Autodesk Fusion 360 part; units mm, degrees
(part 19 of 20)
  spline S762 degree 3 poles (33.1646, -486.3279) (33.0435, -486.3377) (32.8055, -486.3569) (32.6209, -486.5079) (32.5302, -486.582) knots 0 0 0 0 0.035532 0.069798 0.069798 0.069798 0.069798
  spline S763 degree 3 poles (32.5302, -486.582) (32.4569, -486.6887) (32.2898, -486.9318) (32.2821, -487.2288) (32.2779, -487.3954) knots 0 0 0 0 0.038079 0.086792 0.086792 0.086792 0.086792
  line L588 (32.2779, -487.3954) -> (32.2779, -489.4998)
  line L589 (32.2779, -489.4998) -> (31.664, -489.4998)
  line L590 (31.664, -489.4998) -> (31.6639, -487.1464)
  spline S764 degree 3 poles (31.6639, -487.1464) (31.6615, -487.0244) (31.6572, -486.8076) (31.5575, -486.6162) (31.5139, -486.5325) knots 0 0 0 0 0.036008 0.063954 0.063954 0.063954 0.063954
  spline S765 degree 3 poles (31.5139, -486.5325) (31.4516, -486.473) (31.3154, -486.3426) (31.1258, -486.3331) (31.0227, -486.3279) knots 0 0 0 0 0.025037 0.054812 0.054812 0.054812 0.054812
  spline S766 degree 3 poles (31.0227, -486.3279) (30.938, -486.3336) (30.7685, -486.3449) (30.6185, -486.4245) (30.5435, -486.4643) knots 0 0 0 0 0.025173 0.050327 0.050327 0.050327 0.050327
  spline S767 degree 3 poles (30.5435, -486.4643) (30.4749, -486.516) (30.3346, -486.6216) (30.2618, -486.7816) (30.2246, -486.8634) knots 0 0 0 0 0.025339 0.051812 0.051812 0.051812 0.051812
  spline S768 degree 3 poles (30.2246, -486.8634) (30.1959, -486.9697) (30.1291, -487.2172) (30.127, -487.474) (30.1258, -487.6205) knots 0 0 0 0 0.032907 0.076633 0.076633 0.076633 0.076633
  line L591 (30.1258, -487.6205) -> (30.1258, -489.4998)
  line L592 (30.1258, -489.4998) -> (29.5119, -489.4998)
  line L593 (18.0828, -488.1801) -> (18.6967, -488.0982)
  spline S769 degree 3 poles (18.6967, -488.0982) (18.7321, -488.254) (18.7955, -488.533) (18.9765, -488.7531) (19.0565, -488.8503) knots 0 0 0 0 0.04711 0.084389 0.084389 0.084389 0.084389
  spline S770 degree 3 poles (19.0565, -488.8503) (19.1469, -488.9174) (19.3307, -489.054) (19.5593, -489.0716) (19.6756, -489.0805) knots 0 0 0 0 0.033049 0.06726 0.06726 0.06726 0.06726
  spline S771 degree 3 poles (19.6756, -489.0805) (19.814, -489.0683) (20.0891, -489.0441) (20.3016, -488.8679) (20.4071, -488.7803) knots 0 0 0 0 0.040646 0.080767 0.080767 0.080767 0.080767
  spline S772 degree 3 poles (20.4071, -488.7803) (20.4942, -488.6734) (20.6706, -488.4566) (20.6938, -488.1779) (20.7056, -488.0368) knots 0 0 0 0 0.040368 0.081802 0.081802 0.081802 0.081802
  spline S773 degree 3 poles (20.7056, -488.0368) (20.6952, -487.9031) (20.6748, -487.6418) (20.5099, -487.4386) (20.4293, -487.3393) knots 0 0 0 0 0.039196 0.07662 0.07662 0.07662 0.07662
  spline S774 degree 3 poles (20.4293, -487.3393) (20.3292, -487.2593) (20.1239, -487.095) (19.8613, -487.075) (19.7267, -487.0648) knots 0 0 0 0 0.037531 0.077014 0.077014 0.077014 0.077014
  spline S775 degree 3 poles (19.7267, -487.0648) (19.6613, -487.0687) (19.5148, -487.0774) (19.3724, -487.1132) (19.2935, -487.133) knots 0 0 0 0 0.0196 0.043933 0.043933 0.043933 0.043933
  line L594 (19.2935, -487.133) -> (19.3618, -486.5941)
  spline S776 degree 3 poles (19.3618, -486.5941) (19.3802, -486.5961) (19.4131, -486.5996) (19.4462, -486.6005) (19.4607, -486.6009) knots 0 0 0 0 0.005566 0.009918 0.009918 0.009918 0.009918
  spline S777 degree 3 poles (19.4607, -486.6009) (19.5875, -486.5928) (19.838, -486.5768) (20.058, -486.456) (20.1667, -486.3963) knots 0 0 0 0 0.037611 0.074313 0.074313 0.074313 0.074313
  spline S778 degree 3 poles (20.1667, -486.3963) (20.2581, -486.3162) (20.4485, -486.1497) (20.4695, -485.8967) (20.4804, -485.7653) knots 0 0 0 0 0.035073 0.072985 0.072985 0.072985 0.072985
  spline S779 degree 3 poles (20.4804, -485.7653) (20.4716, -485.6582) (20.4541, -485.4476) (20.3186, -485.2856) (20.2519, -485.206) knots 0 0 0 0 0.031391 0.061757 0.061757 0.061757 0.061757
  spline S780 degree 3 poles (20.2519, -485.206) (20.1682, -485.1413) (19.9946, -485.0073) (19.7754, -484.9921) (19.6619, -484.9843) knots 0 0 0 0 0.031011 0.064303 0.064303 0.064303 0.064303
  spline S781 degree 3 poles (19.6619, -484.9843) (19.5485, -484.9927) (19.3271, -485.0092) (19.1509, -485.1438) (19.065, -485.2094) knots 0 0 0 0 0.033306 0.06503 0.06503 0.06503 0.06503
  spline S782 degree 3 poles (19.065, -485.2094) (18.9918, -485.2995) (18.8312, -485.4971) (18.7838, -485.7481) (18.7581, -485.8847) knots 0 0 0 0 0.034298 0.07522 0.07522 0.07522 0.07522
  line L595 (18.7581, -485.8847) -> (18.1441, -485.7756)
  spline S783 degree 3 poles (18.1441, -485.7756) (18.19, -485.5845) (18.2776, -485.2203) (18.5339, -484.9482) (18.6557, -484.8189) knots 0 0 0 0 0.057796 0.110176 0.110176 0.110176 0.110176
  spline S784 degree 3 poles (18.6557, -484.8189) (18.8, -484.7199) (19.0988, -484.515) (19.461, -484.4916) (19.6482, -484.4795) knots 0 0 0 0 0.051494 0.106636 0.106636 0.106636 0.106636
  spline S785 degree 3 poles (19.6482, -484.4795) (19.7811, -484.4864) (20.0429, -484.4999) (20.2835, -484.6039) (20.402, -484.6551) knots 0 0 0 0 0.039552 0.07795 0.07795 0.07795 0.07795
  spline S786 degree 3 poles (20.402, -484.6551) (20.5093, -484.7178) (20.7191, -484.8402) (20.8601, -485.0378) (20.9289, -485.1343) knots 0 0 0 0 0.036811 0.071949 0.071949 0.071949 0.071949
  spline S787 degree 3 poles (20.9289, -485.1343) (20.9821, -485.2365) (21.0875, -485.4388) (21.1035, -485.6663) (21.1114, -485.7789) knots 0 0 0 0 0.034154 0.067635 0.067635 0.067635 0.067635
  spline S788 degree 3 poles (21.1114, -485.7789) (21.1043, -485.8843) (21.0902, -486.0939) (20.9882, -486.2776) (20.9375, -486.369) knots 0 0 0 0 0.031256 0.062193 0.062193 0.062193 0.062193
  spline S789 degree 3 poles (20.9375, -486.369) (20.8702, -486.4542) (20.7295, -486.6323) (20.5278, -486.7372) (20.4225, -486.7919) knots 0 0 0 0 0.032177 0.067318 0.067318 0.067318 0.067318
  spline S790 degree 3 poles (20.4225, -486.7919) (20.5606, -486.8334) (20.8284, -486.9138) (21.0191, -487.1178) (21.1114, -487.2165) knots 0 0 0 0 0.042418 0.082229 0.082229 0.082229 0.082229
  spline S791 degree 3 poles (21.1114, -487.2165) (21.183, -487.3343) (21.3334, -487.5817) (21.3489, -487.8713) (21.357, -488.0231) knots 0 0 0 0 0.040688 0.085491 0.085491 0.085491 0.085491
  spline S792 degree 3 poles (21.357, -488.0231) (21.3369, -488.2333) (21.2967, -488.6544) (21.0188, -488.9735) (20.8795, -489.1333) knots 0 0 0 0 0.061663 0.123588 0.123588 0.123588 0.123588
  spline S793 degree 3 poles (20.8795, -489.1333) (20.7066, -489.2661) (20.3507, -489.5393) (19.9026, -489.5719) (19.6722, -489.5886) knots 0 0 0 0 0.063941 0.131584 0.131584 0.131584 0.131584
  spline S794 degree 3 poles (19.6722, -489.5886) (19.4646, -489.5745) (19.0624, -489.5472) (18.7367, -489.3108) (18.5791, -489.1964) knots 0 0 0 0 0.061033 0.118246 0.118246 0.118246 0.118246
  spline S795 degree 3 poles (18.5791, -489.1964) (18.4495, -489.0541) (18.1853, -488.764) (18.1174, -488.3772) (18.0828, -488.1801) knots 0 0 0 0 0.056507 0.1152 0.1152 0.1152 0.1152
  line L596 (29.5184, -539.499) -> (29.5181, -535.8769)
  line L597 (29.5181, -535.8769) -> (30.0672, -535.8768)
  line L598 (30.0672, -535.8768) -> (30.0672, -536.385)
  spline S796 degree 3 poles (30.0672, -536.385) (30.1291, -536.3004) (30.254, -536.1299) (30.4314, -536.0149) (30.5208, -535.9569) knots 0 0 0 0 0.031158 0.062835 0.062835 0.062835 0.062835
  spline S797 degree 3 poles (30.5208, -535.9569) (30.62, -535.9097) (30.8239, -535.8125) (31.0495, -535.8009) (31.1654, -535.7949) knots 0 0 0 0 0.032617 0.067048 0.067048 0.067048 0.067048
  spline S798 degree 3 poles (31.1654, -535.7949) (31.2899, -535.7996) (31.5223, -535.8084) (31.7293, -535.9133) (31.8254, -535.9619) knots 0 0 0 0 0.036859 0.068796 0.068796 0.068796 0.068796
  spline S799 degree 3 poles (31.8254, -535.9619) (31.9051, -536.0236) (32.066, -536.1483) (32.1475, -536.3349) (32.1887, -536.4291) knots 0 0 0 0 0.029725 0.060035 0.060035 0.060035 0.060035
  spline S800 degree 3 poles (32.1887, -536.4291) (32.3388, -536.2442) (32.6299, -535.8856) (33.0863, -535.8243) (33.3073, -535.7947) knots 0 0 0 0 0.068625 0.133023 0.133023 0.133023 0.133023
  spline S801 degree 3 poles (33.3073, -535.7947) (33.4724, -535.8031) (33.7803, -535.8187) (34.0234, -536.0061) (34.1361, -536.093) knots 0 0 0 0 0.048244 0.08997 0.08997 0.08997 0.08997
  spline S802 degree 3 poles (34.1361, -536.093) (34.2204, -536.2154) (34.4099, -536.4902) (34.4203, -536.8259) (34.4261, -537.0122) knots 0 0 0 0 0.043695 0.098195 0.098195 0.098195 0.098195
  line L599 (34.4261, -537.0122) -> (34.4263, -539.4985)
  line L600 (34.4263, -539.4985) -> (33.8158, -539.4986)
  line L601 (33.8158, -539.4986) -> (33.8156, -537.2169)
  spline S803 degree 3 poles (33.8156, -537.2169) (33.8156, -537.1106) (33.8155, -536.9313) (33.7731, -536.7574) (33.7559, -536.6865) knots 0 0 0 0 0.031711 0.053535 0.053535 0.053535 0.053535
  spline S804 degree 3 poles (33.7559, -536.6865) (33.7314, -536.6348) (33.6816, -536.5294) (33.5873, -536.4607) (33.5393, -536.4256) knots 0 0 0 0 0.016863 0.034394 0.034394 0.034394 0.034394
  spline S805 degree 3 poles (33.5393, -536.4256) (33.4836, -536.3968) (33.3681, -536.337) (33.2381, -536.3303) (33.1709, -536.3267) knots 0 0 0 0 0.018597 0.038532 0.038532 0.038532 0.038532
  spline S806 degree 3 poles (33.1709, -536.3267) (33.0498, -536.3366) (32.8118, -536.3558) (32.6272, -536.5068) (32.5366, -536.5809) knots 0 0 0 0 0.035532 0.069798 0.069798 0.069798 0.069798
  spline S807 degree 3 poles (32.5366, -536.5809) (32.4632, -536.6876) (32.2961, -536.9308) (32.2885, -537.2277) (32.2842, -537.3944) knots 0 0 0 0 0.038079 0.086792 0.086792 0.086792 0.086792
  line L602 (32.2842, -537.3944) -> (32.2844, -539.4987)
  line L603 (32.2844, -539.4987) -> (31.6705, -539.4988)
  line L604 (31.6705, -539.4988) -> (31.6703, -537.1454)
  spline S808 degree 3 poles (31.6703, -537.1454) (31.6679, -537.0234) (31.6636, -536.8066) (31.5638, -536.6152) (31.5202, -536.5315) knots 0 0 0 0 0.036008 0.063954 0.063954 0.063954 0.063954
  spline S809 degree 3 poles (31.5202, -536.5315) (31.458, -536.472) (31.3217, -536.3416) (31.1321, -536.3321) (31.029, -536.3269) knots 0 0 0 0 0.025037 0.054812 0.054812 0.054812 0.054812
  spline S810 degree 3 poles (31.029, -536.3269) (30.9443, -536.3326) (30.7748, -536.344) (30.6248, -536.4236) (30.5499, -536.4634) knots 0 0 0 0 0.025173 0.050327 0.050327 0.050327 0.050327
  spline S811 degree 3 poles (30.5499, -536.4634) (30.4812, -536.5151) (30.3409, -536.6207) (30.2682, -536.7807) (30.231, -536.8625) knots 0 0 0 0 0.025339 0.051812 0.051812 0.051812 0.051812
  spline S812 degree 3 poles (30.231, -536.8625) (30.2023, -536.9688) (30.1355, -537.2163) (30.1334, -537.4731) (30.1321, -537.6196) knots 0 0 0 0 0.032907 0.076633 0.076633 0.076633 0.076633
  line L605 (30.1321, -537.6196) -> (30.1323, -539.4989)
  line L606 (30.1323, -539.4989) -> (29.5184, -539.499)
  line L607 (18.0892, -538.18) -> (18.7031, -538.0981)
  spline S813 degree 3 poles (18.7031, -538.0981) (18.7385, -538.2539) (18.8019, -538.5329) (18.983, -538.7529) (19.063, -538.8501) knots 0 0 0 0 0.04711 0.084389 0.084389 0.084389 0.084389
  spline S814 degree 3 poles (19.063, -538.8501) (19.1534, -538.9173) (19.3372, -539.0539) (19.5658, -539.0714) (19.6821, -539.0803) knots 0 0 0 0 0.033049 0.06726 0.06726 0.06726 0.06726
  spline S815 degree 3 poles (19.6821, -539.0803) (19.8205, -539.0681) (20.0956, -539.0439) (20.3081, -538.8676) (20.4136, -538.7801) knots 0 0 0 0 0.040646 0.080767 0.080767 0.080767 0.080767
  spline S816 degree 3 poles (20.4136, -538.7801) (20.5007, -538.6731) (20.677, -538.4564) (20.7002, -538.1777) (20.712, -538.0365) knots 0 0 0 0 0.040368 0.081802 0.081802 0.081802 0.081802
  spline S817 degree 3 poles (20.712, -538.0365) (20.7016, -537.9029) (20.6812, -537.6416) (20.5162, -537.4384) (20.4357, -537.3391) knots 0 0 0 0 0.039196 0.07662 0.07662 0.07662 0.07662
  spline S818 degree 3 poles (20.4357, -537.3391) (20.3356, -537.259) (20.1303, -537.0948) (19.8677, -537.0748) (19.7331, -537.0646) knots 0 0 0 0 0.037531 0.077014 0.077014 0.077014 0.077014
  spline S819 degree 3 poles (19.7331, -537.0646) (19.6677, -537.0685) (19.5212, -537.0772) (19.3788, -537.113) (19.2999, -537.1328) knots 0 0 0 0 0.0196 0.043933 0.043933 0.043933 0.043933
  line L608 (19.2999, -537.1328) -> (19.3681, -536.594)
  spline S820 degree 3 poles (19.3681, -536.594) (19.3865, -536.5959) (19.4194, -536.5995) (19.4525, -536.6004) (19.467, -536.6008) knots 0 0 0 0 0.005566 0.009918 0.009918 0.009918 0.009918
  spline S821 degree 3 poles (19.467, -536.6008) (19.5938, -536.5927) (19.8444, -536.5766) (20.0643, -536.4558) (20.173, -536.3961) knots 0 0 0 0 0.037611 0.074313 0.074313 0.074313 0.074313
  spline S822 degree 3 poles (20.173, -536.3961) (20.2644, -536.316) (20.4548, -536.1495) (20.4758, -535.8965) (20.4867, -535.7651) knots 0 0 0 0 0.035073 0.072985 0.072985 0.072985 0.072985
  spline S823 degree 3 poles (20.4867, -535.7651) (20.4778, -535.658) (20.4603, -535.4473) (20.3248, -535.2854) (20.2581, -535.2058) knots 0 0 0 0 0.031391 0.061757 0.061757 0.061757 0.061757
  spline S824 degree 3 poles (20.2581, -535.2058) (20.1744, -535.1411) (20.0008, -535.0071) (19.7816, -534.992) (19.6681, -534.9841) knots 0 0 0 0 0.031011 0.064303 0.064303 0.064303 0.064303
  spline S825 degree 3 poles (19.6681, -534.9841) (19.5547, -534.9926) (19.3333, -535.009) (19.1572, -535.1436) (19.0712, -535.2093) knots 0 0 0 0 0.033306 0.06503 0.06503 0.06503 0.06503
  spline S826 degree 3 poles (19.0712, -535.2093) (18.998, -535.2994) (18.8375, -535.4969) (18.7901, -535.748) (18.7643, -535.8846) knots 0 0 0 0 0.034298 0.07522 0.07522 0.07522 0.07522
  line L609 (18.7643, -535.8846) -> (18.1504, -535.7755)
  spline S827 degree 3 poles (18.1504, -535.7755) (18.1963, -535.5844) (18.2838, -535.2202) (18.5401, -534.9481) (18.6619, -534.8188) knots 0 0 0 0 0.057796 0.110176 0.110176 0.110176 0.110176
  spline S828 degree 3 poles (18.6619, -534.8188) (18.8062, -534.7198) (19.105, -534.5149) (19.4671, -534.4915) (19.6544, -534.4793) knots 0 0 0 0 0.051494 0.106636 0.106636 0.106636 0.106636
  spline S829 degree 3 poles (19.6544, -534.4793) (19.7872, -534.4862) (20.0491, -534.4997) (20.2896, -534.6037) (20.4082, -534.6549) knots 0 0 0 0 0.039552 0.07795 0.07795 0.07795 0.07795
  spline S830 degree 3 poles (20.4082, -534.6549) (20.5155, -534.7176) (20.7253, -534.84) (20.8663, -535.0376) (20.9351, -535.1341) knots 0 0 0 0 0.036811 0.071949 0.071949 0.071949 0.071949
  spline S831 degree 3 poles (20.9351, -535.1341) (20.9884, -535.2362) (21.0938, -535.4385) (21.1098, -535.6661) (21.1177, -535.7787) knots 0 0 0 0 0.034154 0.067635 0.067635 0.067635 0.067635
  spline S832 degree 3 poles (21.1177, -535.7787) (21.1106, -535.884) (21.0965, -536.0937) (20.9945, -536.2774) (20.9438, -536.3687) knots 0 0 0 0 0.031256 0.062193 0.062193 0.062193 0.062193
  spline S833 degree 3 poles (20.9438, -536.3687) (20.8765, -536.4539) (20.7358, -536.6321) (20.5341, -536.7369) (20.4288, -536.7917) knots 0 0 0 0 0.032177 0.067318 0.067318 0.067318 0.067318
  spline S834 degree 3 poles (20.4288, -536.7917) (20.567, -536.8332) (20.8348, -536.9135) (21.0255, -537.1175) (21.1178, -537.2163) knots 0 0 0 0 0.042418 0.082229 0.082229 0.082229 0.082229
  spline S835 degree 3 poles (21.1178, -537.2163) (21.1894, -537.334) (21.3398, -537.5814) (21.3553, -537.871) (21.3634, -538.0228) knots 0 0 0 0 0.040688 0.085491 0.085491 0.085491 0.085491
  spline S836 degree 3 poles (21.3634, -538.0228) (21.3434, -538.233) (21.3032, -538.6541) (21.0253, -538.9732) (20.886, -539.1331) knots 0 0 0 0 0.061663 0.123588 0.123588 0.123588 0.123588
  spline S837 degree 3 poles (20.886, -539.1331) (20.7131, -539.2658) (20.3573, -539.5391) (19.9091, -539.5717) (19.6787, -539.5885) knots 0 0 0 0 0.063941 0.131584 0.131584 0.131584 0.131584
  spline S838 degree 3 poles (19.6787, -539.5885) (19.4711, -539.5744) (19.0689, -539.547) (18.7432, -539.3107) (18.5856, -539.1963) knots 0 0 0 0 0.061033 0.118246 0.118246 0.118246 0.118246
  spline S839 degree 3 poles (18.5856, -539.1963) (18.456, -539.054) (18.1918, -538.7639) (18.1238, -538.3771) (18.0892, -538.18) knots 0 0 0 0 0.056507 0.1152 0.1152 0.1152 0.1152
  line L610 (29.5554, -589.4999) -> (29.5554, -585.8778)
  line L611 (29.5554, -585.8778) -> (30.1045, -585.8778)
  line L612 (30.1045, -585.8778) -> (30.1045, -586.386)
  spline S840 degree 3 poles (30.1045, -586.386) (30.1664, -586.3014) (30.2913, -586.1309) (30.4687, -586.0159) (30.5581, -585.958) knots 0 0 0 0 0.031158 0.062835 0.062835 0.062835 0.062835
  spline S841 degree 3 poles (30.5581, -585.958) (30.6573, -585.9107) (30.8612, -585.8136) (31.0868, -585.802) (31.2027, -585.796) knots 0 0 0 0 0.032617 0.067048 0.067048 0.067048 0.067048
  spline S842 degree 3 poles (31.2027, -585.796) (31.3272, -585.8007) (31.5596, -585.8095) (31.7666, -585.9144) (31.8627, -585.9631) knots 0 0 0 0 0.036859 0.068796 0.068796 0.068796 0.068796
  spline S843 degree 3 poles (31.8627, -585.9631) (31.9424, -586.0248) (32.1033, -586.1495) (32.1848, -586.3361) (32.2259, -586.4303) knots 0 0 0 0 0.029725 0.060035 0.060035 0.060035 0.060035
  spline S844 degree 3 poles (32.2259, -586.4303) (32.3761, -586.2454) (32.6672, -585.8868) (33.1236, -585.8256) (33.3446, -585.796) knots 0 0 0 0 0.068625 0.133023 0.133023 0.133023 0.133023
  spline S845 degree 3 poles (33.3446, -585.796) (33.5097, -585.8044) (33.8176, -585.82) (34.0607, -586.0075) (34.1734, -586.0944) knots 0 0 0 0 0.048244 0.08997 0.08997 0.08997 0.08997
  spline S846 degree 3 poles (34.1734, -586.0944) (34.2577, -586.2167) (34.4471, -586.4916) (34.4575, -586.8273) (34.4633, -587.0135) knots 0 0 0 0 0.043695 0.098195 0.098195 0.098195 0.098195
  line L613 (34.4633, -587.0135) -> (34.4633, -589.4999)
  line L614 (34.4633, -589.4999) -> (33.8528, -589.4999)
  line L615 (33.8528, -589.4999) -> (33.8528, -587.2182)
  spline S847 degree 3 poles (33.8528, -587.2182) (33.8528, -587.112) (33.8527, -586.9327) (33.8104, -586.7587) (33.7931, -586.6878) knots 0 0 0 0 0.031711 0.053535 0.053535 0.053535 0.053535
  spline S848 degree 3 poles (33.7931, -586.6878) (33.7687, -586.6362) (33.7188, -586.5308) (33.6246, -586.462) (33.5765, -586.4269) knots 0 0 0 0 0.016863 0.034394 0.034394 0.034394 0.034394
  spline S849 degree 3 poles (33.5765, -586.4269) (33.5208, -586.3981) (33.4054, -586.3383) (33.2754, -586.3315) (33.2082, -586.328) knots 0 0 0 0 0.018597 0.038532 0.038532 0.038532 0.038532
  spline S850 degree 3 poles (33.2082, -586.328) (33.087, -586.3378) (32.8491, -586.3571) (32.6644, -586.508) (32.5738, -586.5821) knots 0 0 0 0 0.035532 0.069798 0.069798 0.069798 0.069798
  spline S851 degree 3 poles (32.5738, -586.5821) (32.5005, -586.6888) (32.3333, -586.932) (32.3257, -587.2289) (32.3214, -587.3955) knots 0 0 0 0 0.038079 0.086792 0.086792 0.086792 0.086792
  line L616 (32.3214, -587.3955) -> (32.3214, -589.4999)
  line L617 (32.3214, -589.4999) -> (31.7075, -589.4999)
  line L618 (31.7075, -589.4999) -> (31.7075, -587.1466)
  spline S852 degree 3 poles (31.7075, -587.1466) (31.7051, -587.0245) (31.7008, -586.8077) (31.601, -586.6163) (31.5574, -586.5327) knots 0 0 0 0 0.036008 0.063954 0.063954 0.063954 0.063954
  spline S853 degree 3 poles (31.5574, -586.5327) (31.4952, -586.4731) (31.359, -586.3427) (31.1693, -586.3332) (31.0663, -586.328) knots 0 0 0 0 0.025037 0.054812 0.054812 0.054812 0.054812
  spline S854 degree 3 poles (31.0663, -586.328) (30.9815, -586.3337) (30.8121, -586.345) (30.6621, -586.4247) (30.5871, -586.4645) knots 0 0 0 0 0.025172 0.050327 0.050327 0.050327 0.050327
  spline S855 degree 3 poles (30.5871, -586.4645) (30.5185, -586.5161) (30.3782, -586.6217) (30.3054, -586.7817) (30.2682, -586.8635) knots 0 0 0 0 0.025339 0.051812 0.051812 0.051812 0.051812
  spline S856 degree 3 poles (30.2682, -586.8635) (30.2395, -586.9698) (30.1727, -587.2173) (30.1705, -587.4741) (30.1693, -587.6207) knots 0 0 0 0 0.032907 0.076633 0.076633 0.076633 0.076633
  line L619 (30.1693, -587.6207) -> (30.1693, -589.4999)
  line L620 (30.1693, -589.4999) -> (29.5554, -589.4999)
  line L621 (21.3494, -588.9099) -> (21.3494, -589.5)
  line L622 (21.3494, -589.5) -> (18.0445, -589.5)
  spline S857 degree 3 poles (18.0445, -589.5) (18.0457, -589.4269) (18.0482, -589.2812) (18.0935, -589.1427) (18.1161, -589.0737) knots 0 0 0 0 0.021791 0.043448 0.043448 0.043448 0.043448
  spline S858 degree 3 poles (18.1161, -589.0737) (18.1664, -588.9593) (18.2717, -588.7199) (18.435, -588.5154) (18.5203, -588.4086) knots 0 0 0 0 0.037314 0.078118 0.078118 0.078118 0.078118
  spline S859 degree 3 poles (18.5203, -588.4086) (18.6313, -588.2886) (18.8818, -588.0181) (19.1656, -587.7825) (19.3235, -587.6514) knots 0 0 0 0 0.048996 0.110487 0.110487 0.110487 0.110487
  spline S860 degree 3 poles (19.3235, -587.6514) (19.5582, -587.459) (19.9537, -587.1347) (20.2889, -586.7491) (20.4251, -586.5924) knots 0 0 0 0 0.090844 0.153043 0.153043 0.153043 0.153043
  spline S861 degree 3 poles (20.4251, -586.5924) (20.5085, -586.4701) (20.6616, -586.2455) (20.696, -585.9766) (20.7116, -585.854) knots 0 0 0 0 0.043642 0.080205 0.080205 0.080205 0.080205
  spline S862 degree 3 poles (20.7116, -585.854) (20.7008, -585.7372) (20.6793, -585.5042) (20.5268, -585.3268) (20.4507, -585.2384) knots 0 0 0 0 0.034264 0.068363 0.068363 0.068363 0.068363
  spline S863 degree 3 poles (20.4507, -585.2384) (20.3544, -585.1653) (20.1536, -585.0129) (19.9015, -584.9963) (19.7702, -584.9877) knots 0 0 0 0 0.035452 0.073952 0.073952 0.073952 0.073952
  spline S864 degree 3 poles (19.7702, -584.9877) (19.6321, -584.9966) (19.368, -585.0136) (19.16, -585.1762) (19.0608, -585.2537) knots 0 0 0 0 0.040455 0.077352 0.077352 0.077352 0.077352
  spline S865 degree 3 poles (19.0608, -585.2537) (18.9832, -585.3553) (18.8174, -585.572) (18.8004, -585.8453) (18.7914, -585.9904) knots 0 0 0 0 0.037518 0.080034 0.080034 0.080034 0.080034
  line L623 (18.7914, -585.9904) -> (18.1604, -585.9256)
  spline S866 degree 3 poles (18.1604, -585.9256) (18.1919, -585.7089) (18.2511, -585.3018) (18.5216, -584.9937) (18.6481, -584.8496) knots 0 0 0 0 0.064088 0.120417 0.120417 0.120417 0.120417
  spline S867 degree 3 poles (18.6481, -584.8496) (18.8081, -584.7418) (19.1503, -584.5111) (19.5637, -584.4905) (19.7839, -584.4795) knots 0 0 0 0 0.056784 0.121484 0.121484 0.121484 0.121484
  spline S868 degree 3 poles (19.7839, -584.4795) (20.0064, -584.4917) (20.4261, -584.5148) (20.7642, -584.7623) (20.923, -584.8786) knots 0 0 0 0 0.065229 0.123034 0.123034 0.123034 0.123034
  spline S869 degree 3 poles (20.923, -584.8786) (21.0454, -585.02) (21.2914, -585.3046) (21.3255, -585.6793) (21.3426, -585.8676) knots 0 0 0 0 0.054646 0.10988 0.10988 0.10988 0.10988
  spline S870 degree 3 poles (21.3426, -585.8676) (21.3372, -585.9678) (21.3263, -586.1707) (21.2556, -586.3612) (21.2198, -586.4577) knots 0 0 0 0 0.029916 0.060578 0.060578 0.060578 0.060578
  spline S871 degree 3 poles (21.2198, -586.4577) (21.1689, -586.5592) (21.0584, -586.7794) (20.8984, -586.967) (20.8122, -587.0682) knots 0 0 0 0 0.033943 0.073642 0.073642 0.073642 0.073642
  spline S872 degree 3 poles (20.8122, -587.0682) (20.6875, -587.1967) (20.3873, -587.5062) (20.0582, -587.7851) (19.8658, -587.9481) knots 0 0 0 0 0.05369 0.129298 0.129298 0.129298 0.129298
  spline S873 degree 3 poles (19.8658, -587.9481) (19.7127, -588.0758) (19.4698, -588.2784) (19.241, -588.4967) (19.1563, -588.5774) knots 0 0 0 0 0.059772 0.09485 0.09485 0.09485 0.09485
  spline S874 degree 3 poles (19.1563, -588.5774) (19.107, -588.6315) (19.012, -588.7356) (18.9345, -588.8533) (18.8971, -588.9099) knots 0 0 0 0 0.021914 0.042221 0.042221 0.042221 0.042221
  line L624 (18.8971, -588.9099) -> (21.3494, -588.9099)
  line L625 (29.5579, -639.4997) -> (29.5578, -635.8776)
  line L626 (29.5578, -635.8776) -> (30.1069, -635.8775)
  line L627 (30.1069, -635.8775) -> (30.1069, -636.3857)
  spline S875 degree 3 poles (30.1069, -636.3857) (30.1688, -636.3012) (30.2937, -636.1306) (30.4711, -636.0156) (30.5605, -635.9577) knots 0 0 0 0 0.031158 0.062835 0.062835 0.062835 0.062835
  spline S876 degree 3 poles (30.5605, -635.9577) (30.6597, -635.9104) (30.8636, -635.8133) (31.0892, -635.8016) (31.2051, -635.7956) knots 0 0 0 0 0.032617 0.067048 0.067048 0.067048 0.067048
  spline S877 degree 3 poles (31.2051, -635.7956) (31.3296, -635.8004) (31.562, -635.8092) (31.769, -635.9141) (31.8651, -635.9628) knots 0 0 0 0 0.036859 0.068796 0.068796 0.068796 0.068796
  spline S878 degree 3 poles (31.8651, -635.9628) (31.9448, -636.0245) (32.1057, -636.1491) (32.1872, -636.3358) (32.2283, -636.43) knots 0 0 0 0 0.029725 0.060035 0.060035 0.060035 0.060035
  spline S879 degree 3 poles (32.2283, -636.43) (32.3785, -636.245) (32.6696, -635.8865) (33.126, -635.8252) (33.347, -635.7956) knots 0 0 0 0 0.068625 0.133023 0.133023 0.133023 0.133023
  spline S880 degree 3 poles (33.347, -635.7956) (33.5121, -635.804) (33.82, -635.8197) (34.0631, -636.0071) (34.1758, -636.094) knots 0 0 0 0 0.048244 0.08997 0.08997 0.08997 0.08997
  spline S881 degree 3 poles (34.1758, -636.094) (34.2601, -636.2163) (34.4495, -636.4912) (34.4599, -636.8269) (34.4657, -637.0132) knots 0 0 0 0 0.043695 0.098195 0.098195 0.098195 0.098195
  line L628 (34.4657, -637.0132) -> (34.4658, -639.4995)
  line L629 (34.4658, -639.4995) -> (33.8553, -639.4995)
  line L630 (33.8553, -639.4995) -> (33.8552, -637.2178)
  spline S882 degree 3 poles (33.8552, -637.2178) (33.8552, -637.1116) (33.8552, -636.9323) (33.8128, -636.7584) (33.7955, -636.6875) knots 0 0 0 0 0.031711 0.053535 0.053535 0.053535 0.053535
  spline S883 degree 3 poles (33.7955, -636.6875) (33.7711, -636.6358) (33.7212, -636.5304) (33.627, -636.4616) (33.5789, -636.4266) knots 0 0 0 0 0.016863 0.034394 0.034394 0.034394 0.034394
  spline S884 degree 3 poles (33.5789, -636.4266) (33.5232, -636.3977) (33.4078, -636.338) (33.2778, -636.3312) (33.2106, -636.3277) knots 0 0 0 0 0.018597 0.038532 0.038532 0.038532 0.038532
  spline S885 degree 3 poles (33.2106, -636.3277) (33.0895, -636.3375) (32.8515, -636.3567) (32.6669, -636.5077) (32.5762, -636.5818) knots 0 0 0 0 0.035532 0.069798 0.069798 0.069798 0.069798
  spline S886 degree 3 poles (32.5762, -636.5818) (32.5029, -636.6885) (32.3358, -636.9316) (32.3281, -637.2286) (32.3239, -637.3952) knots 0 0 0 0 0.038079 0.086792 0.086792 0.086792 0.086792
  line L631 (32.3239, -637.3952) -> (32.3239, -639.4996)
  line L632 (32.3239, -639.4996) -> (31.71, -639.4996)
  line L633 (31.71, -639.4996) -> (31.7099, -637.1462)
  spline S887 degree 3 poles (31.7099, -637.1462) (31.7075, -637.0242) (31.7032, -636.8074) (31.6034, -636.616) (31.5598, -636.5323) knots 0 0 0 0 0.036008 0.063954 0.063954 0.063954 0.063954
  spline S888 degree 3 poles (31.5598, -636.5323) (31.4976, -636.4728) (31.3614, -636.3424) (31.1717, -636.3329) (31.0687, -636.3277) knots 0 0 0 0 0.025037 0.054812 0.054812 0.054812 0.054812
  spline S889 degree 3 poles (31.0687, -636.3277) (30.984, -636.3334) (30.8145, -636.3447) (30.6645, -636.4244) (30.5895, -636.4642) knots 0 0 0 0 0.025172 0.050327 0.050327 0.050327 0.050327
  spline S890 degree 3 poles (30.5895, -636.4642) (30.5209, -636.5158) (30.3806, -636.6214) (30.3078, -636.7814) (30.2706, -636.8632) knots 0 0 0 0 0.025339 0.051812 0.051812 0.051812 0.051812
  spline S891 degree 3 poles (30.2706, -636.8632) (30.2419, -636.9695) (30.1751, -637.2171) (30.173, -637.4738) (30.1717, -637.6204) knots 0 0 0 0 0.032907 0.076633 0.076633 0.076633 0.076633
  line L634 (30.1717, -637.6204) -> (30.1718, -639.4996)
  line L635 (30.1718, -639.4996) -> (29.5579, -639.4997)
  line L636 (21.3519, -638.9098) -> (21.3519, -639.4999)
  line L637 (21.3519, -639.4999) -> (18.047, -639.5)
  spline S892 degree 3 poles (18.047, -639.5) (18.0482, -639.4269) (18.0507, -639.2812) (18.096, -639.1427) (18.1186, -639.0736) knots 0 0 0 0 0.021791 0.043448 0.043448 0.043448 0.043448
  spline S893 degree 3 poles (18.1186, -639.0736) (18.1689, -638.9593) (18.2742, -638.7199) (18.4374, -638.5154) (18.5227, -638.4086) knots 0 0 0 0 0.037314 0.078118 0.078118 0.078118 0.078118
  spline S894 degree 3 poles (18.5227, -638.4086) (18.6338, -638.2886) (18.8843, -638.0181) (19.168, -637.7825) (19.3259, -637.6514) knots 0 0 0 0 0.048996 0.110487 0.110487 0.110487 0.110487
  spline S895 degree 3 poles (19.3259, -637.6514) (19.5606, -637.4589) (19.9561, -637.1347) (20.2913, -636.7491) (20.4275, -636.5923) knots 0 0 0 0 0.090844 0.153043 0.153043 0.153043 0.153043
  spline S896 degree 3 poles (20.4275, -636.5923) (20.5109, -636.4701) (20.6641, -636.2454) (20.6984, -635.9765) (20.714, -635.8539) knots 0 0 0 0 0.043642 0.080205 0.080205 0.080205 0.080205
  spline S897 degree 3 poles (20.714, -635.8539) (20.7032, -635.7371) (20.6817, -635.5041) (20.5292, -635.3268) (20.4531, -635.2383) knots 0 0 0 0 0.034264 0.068363 0.068363 0.068363 0.068363
  spline S898 degree 3 poles (20.4531, -635.2383) (20.3568, -635.1652) (20.156, -635.0128) (19.9039, -634.9963) (19.7726, -634.9876) knots 0 0 0 0 0.035452 0.073952 0.073952 0.073952 0.073952
  spline S899 degree 3 poles (19.7726, -634.9876) (19.6345, -634.9965) (19.3704, -635.0136) (19.1624, -635.1761) (19.0632, -635.2537) knots 0 0 0 0 0.040455 0.077352 0.077352 0.077352 0.077352
  spline S900 degree 3 poles (19.0632, -635.2537) (18.9855, -635.3553) (18.8198, -635.572) (18.8028, -635.8452) (18.7938, -635.9904) knots 0 0 0 0 0.037518 0.080034 0.080034 0.080034 0.080034
  line L638 (18.7938, -635.9904) -> (18.1628, -635.9256)
  spline S901 degree 3 poles (18.1628, -635.9256) (18.1943, -635.7089) (18.2535, -635.3018) (18.524, -634.9937) (18.6505, -634.8495) knots 0 0 0 0 0.064088 0.120417 0.120417 0.120417 0.120417
  spline S902 degree 3 poles (18.6505, -634.8495) (18.8105, -634.7417) (19.1526, -634.5111) (19.5661, -634.4904) (19.7863, -634.4795) knots 0 0 0 0 0.056784 0.121484 0.121484 0.121484 0.121484
  spline S903 degree 3 poles (19.7863, -634.4795) (20.0088, -634.4917) (20.4285, -634.5147) (20.7666, -634.7622) (20.9254, -634.8785) knots 0 0 0 0 0.065229 0.123034 0.123034 0.123034 0.123034
  spline S904 degree 3 poles (20.9254, -634.8785) (21.0478, -635.02) (21.2938, -635.3045) (21.3278, -635.6792) (21.345, -635.8675) knots 0 0 0 0 0.054646 0.10988 0.10988 0.10988 0.10988
  spline S905 degree 3 poles (21.345, -635.8675) (21.3396, -635.9677) (21.3287, -636.1706) (21.258, -636.3612) (21.2222, -636.4576) knots 0 0 0 0 0.029916 0.060578 0.060578 0.060578 0.060578
  spline S906 degree 3 poles (21.2222, -636.4576) (21.1713, -636.5591) (21.0608, -636.7793) (20.9009, -636.9669) (20.8146, -637.0681) knots 0 0 0 0 0.033943 0.073642 0.073642 0.073642 0.073642
  spline S907 degree 3 poles (20.8146, -637.0681) (20.69, -637.1966) (20.3897, -637.5062) (20.0606, -637.785) (19.8682, -637.9481) knots 0 0 0 0 0.05369 0.129298 0.129298 0.129298 0.129298
  spline S908 degree 3 poles (19.8682, -637.9481) (19.7151, -638.0758) (19.4723, -638.2784) (19.2434, -638.4966) (19.1588, -638.5774) knots 0 0 0 0 0.059772 0.09485 0.09485 0.09485 0.09485
  spline S909 degree 3 poles (19.1588, -638.5774) (19.1095, -638.6314) (19.0145, -638.7356) (18.9369, -638.8533) (18.8996, -638.9099) knots 0 0 0 0 0.021914 0.042221 0.042221 0.042221 0.042221
  line L639 (18.8996, -638.9099) -> (21.3519, -638.9098)
  line L640 (29.2783, -689.4998) -> (29.2783, -685.8777)
  line L641 (29.2783, -685.8777) -> (29.8274, -685.8777)
  line L642 (29.8274, -685.8777) -> (29.8274, -686.3859)
  spline S910 degree 3 poles (29.8274, -686.3859) (29.8893, -686.3014) (30.0142, -686.1308) (30.1916, -686.0158) (30.281, -685.9579) knots 0 0 0 0 0.031158 0.062835 0.062835 0.062835 0.062835
  spline S911 degree 3 poles (30.281, -685.9579) (30.3802, -685.9106) (30.5841, -685.8135) (30.8097, -685.8019) (30.9256, -685.7959) knots 0 0 0 0 0.032617 0.067048 0.067048 0.067048 0.067048
  spline S912 degree 3 poles (30.9256, -685.7959) (31.0501, -685.8006) (31.2825, -685.8095) (31.4895, -685.9143) (31.5856, -685.963) knots 0 0 0 0 0.036859 0.068796 0.068796 0.068796 0.068796
  spline S913 degree 3 poles (31.5856, -685.963) (31.6652, -686.0247) (31.8262, -686.1494) (31.9077, -686.336) (31.9488, -686.4302) knots 0 0 0 0 0.029725 0.060035 0.060035 0.060035 0.060035
  spline S914 degree 3 poles (31.9488, -686.4302) (32.099, -686.2453) (32.3901, -685.8867) (32.8465, -685.8255) (33.0675, -685.7958) knots 0 0 0 0 0.068625 0.133023 0.133023 0.133023 0.133023
  spline S915 degree 3 poles (33.0675, -685.7958) (33.2326, -685.8042) (33.5405, -685.8199) (33.7835, -686.0073) (33.8963, -686.0943) knots 0 0 0 0 0.048244 0.08997 0.08997 0.08997 0.08997
  spline S916 degree 3 poles (33.8963, -686.0943) (33.9806, -686.2166) (34.17, -686.4915) (34.1804, -686.8271) (34.1862, -687.0134) knots 0 0 0 0 0.043695 0.098195 0.098195 0.098195 0.098195
  line L643 (34.1862, -687.0134) -> (34.1862, -689.4998)
  line L644 (34.1862, -689.4998) -> (33.5757, -689.4998)
  line L645 (33.5757, -689.4998) -> (33.5757, -687.2181)
  spline S917 degree 3 poles (33.5757, -687.2181) (33.5757, -687.1119) (33.5756, -686.9325) (33.5333, -686.7586) (33.516, -686.6877) knots 0 0 0 0 0.031711 0.053535 0.053535 0.053535 0.053535
  spline S918 degree 3 poles (33.516, -686.6877) (33.4916, -686.636) (33.4417, -686.5306) (33.3475, -686.4619) (33.2994, -686.4268) knots 0 0 0 0 0.016863 0.034394 0.034394 0.034394 0.034394
  spline S919 degree 3 poles (33.2994, -686.4268) (33.2437, -686.398) (33.1283, -686.3382) (32.9983, -686.3314) (32.9311, -686.3279) knots 0 0 0 0 0.018597 0.038532 0.038532 0.038532 0.038532
  spline S920 degree 3 poles (32.9311, -686.3279) (32.8099, -686.3377) (32.572, -686.357) (32.3873, -686.5079) (32.2967, -686.582) knots 0 0 0 0 0.035532 0.069798 0.069798 0.069798 0.069798
  spline S921 degree 3 poles (32.2967, -686.582) (32.2234, -686.6887) (32.0562, -686.9319) (32.0486, -687.2288) (32.0443, -687.3954) knots 0 0 0 0 0.038079 0.086792 0.086792 0.086792 0.086792
  line L646 (32.0443, -687.3954) -> (32.0443, -689.4998)
  line L647 (32.0443, -689.4998) -> (31.4304, -689.4998)
  line L648 (31.4304, -689.4998) -> (31.4304, -687.1465)
  spline S922 degree 3 poles (31.4304, -687.1465) (31.428, -687.0244) (31.4237, -686.8076) (31.3239, -686.6162) (31.2803, -686.5326) knots 0 0 0 0 0.036008 0.063954 0.063954 0.063954 0.063954
  spline S923 degree 3 poles (31.2803, -686.5326) (31.2181, -686.473) (31.0819, -686.3426) (30.8922, -686.3331) (30.7892, -686.3279) knots 0 0 0 0 0.025037 0.054812 0.054812 0.054812 0.054812
  spline S924 degree 3 poles (30.7892, -686.3279) (30.7044, -686.3336) (30.535, -686.345) (30.385, -686.4246) (30.31, -686.4644) knots 0 0 0 0 0.025173 0.050327 0.050327 0.050327 0.050327
  spline S925 degree 3 poles (30.31, -686.4644) (30.2414, -686.516) (30.1011, -686.6216) (30.0283, -686.7817) (29.9911, -686.8634) knots 0 0 0 0 0.025339 0.051812 0.051812 0.051812 0.051812
  spline S926 degree 3 poles (29.9911, -686.8634) (29.9624, -686.9697) (29.8956, -687.2173) (29.8934, -687.474) (29.8922, -687.6206) knots 0 0 0 0 0.032907 0.076633 0.076633 0.076633 0.076633
  line L649 (29.8922, -687.6206) -> (29.8922, -689.4998)
  line L650 (29.8922, -689.4998) -> (29.2783, -689.4998)
  line L651 (20.1583, -689.5) -> (19.5443, -689.5)
  line L652 (19.5443, -689.5) -> (19.5443, -685.588)
  spline S927 degree 3 poles (19.5443, -685.588) (19.4606, -685.6608) (19.2792, -685.8187) (19.0736, -685.9436) (18.9628, -686.0109) knots 0 0 0 0 0.033221 0.072019 0.072019 0.072019 0.072019
  spline S928 degree 3 poles (18.9628, -686.0109) (18.8503, -686.0753) (18.6416, -686.1948) (18.4191, -686.286) (18.3165, -686.3281) knots 0 0 0 0 0.03884 0.072064 0.072064 0.072064 0.072064
  line L653 (18.3165, -686.3281) -> (18.3165, -685.7346)
  spline S929 degree 3 poles (18.3165, -685.7346) (18.4811, -685.6511) (18.8025, -685.4881) (19.081, -685.2595) (19.2169, -685.148) knots 0 0 0 0 0.05519 0.10775 0.10775 0.10775 0.10775
  spline S930 degree 3 poles (19.2169, -685.148) (19.3329, -685.0399) (19.5456, -684.8418) (19.6947, -684.5927) (19.7626, -684.4795) knots 0 0 0 0 0.047275 0.086674 0.086674 0.086674 0.086674
  line L654 (19.7626, -684.4795) -> (20.1582, -684.4795)
  line L655 (20.1582, -684.4795) -> (20.1583, -689.5)
  line L656 (29.2799, -739.4997) -> (29.2798, -735.8776)
  line L657 (29.2798, -735.8776) -> (29.8289, -735.8776)
  line L658 (29.8289, -735.8776) -> (29.8289, -736.3858)
  spline S931 degree 3 poles (29.8289, -736.3858) (29.8908, -736.3012) (30.0157, -736.1307) (30.1931, -736.0157) (30.2825, -735.9577) knots 0 0 0 0 0.031158 0.062835 0.062835 0.062835 0.062835
  spline S932 degree 3 poles (30.2825, -735.9577) (30.3817, -735.9105) (30.5856, -735.8134) (30.8112, -735.8017) (30.9271, -735.7957) knots 0 0 0 0 0.032617 0.067048 0.067048 0.067048 0.067048
  spline S933 degree 3 poles (30.9271, -735.7957) (31.0516, -735.8004) (31.284, -735.8093) (31.491, -735.9141) (31.5871, -735.9628) knots 0 0 0 0 0.036859 0.068796 0.068796 0.068796 0.068796
  spline S934 degree 3 poles (31.5871, -735.9628) (31.6668, -736.0245) (31.8277, -736.1492) (31.9092, -736.3358) (31.9503, -736.4301) knots 0 0 0 0 0.029725 0.060035 0.060035 0.060035 0.060035
  spline S935 degree 3 poles (31.9503, -736.4301) (32.1005, -736.2451) (32.3916, -735.8865) (32.848, -735.8253) (33.069, -735.7957) knots 0 0 0 0 0.068625 0.133023 0.133023 0.133023 0.133023
  spline S936 degree 3 poles (33.069, -735.7957) (33.2341, -735.8041) (33.542, -735.8197) (33.7851, -736.0072) (33.8978, -736.0941) knots 0 0 0 0 0.048244 0.08997 0.08997 0.08997 0.08997
  spline S937 degree 3 poles (33.8978, -736.0941) (33.9821, -736.2164) (34.1715, -736.4913) (34.1819, -736.8269) (34.1877, -737.0132) knots 0 0 0 0 0.043695 0.098195 0.098195 0.098195 0.098195
  line L659 (34.1877, -737.0132) -> (34.1878, -739.4996)
  line L660 (34.1878, -739.4996) -> (33.5773, -739.4996)
  line L661 (33.5773, -739.4996) -> (33.5772, -737.2179)
  spline S938 degree 3 poles (33.5772, -737.2179) (33.5772, -737.1117) (33.5772, -736.9323) (33.5348, -736.7584) (33.5175, -736.6875) knots 0 0 0 0 0.031711 0.053535 0.053535 0.053535 0.053535
  spline S939 degree 3 poles (33.5175, -736.6875) (33.4931, -736.6359) (33.4432, -736.5305) (33.349, -736.4617) (33.3009, -736.4266) knots 0 0 0 0 0.016863 0.034394 0.034394 0.034394 0.034394
  spline S940 degree 3 poles (33.3009, -736.4266) (33.2452, -736.3978) (33.1298, -736.338) (32.9998, -736.3312) (32.9326, -736.3277) knots 0 0 0 0 0.018597 0.038532 0.038532 0.038532 0.038532
  spline S941 degree 3 poles (32.9326, -736.3277) (32.8115, -736.3375) (32.5735, -736.3568) (32.3889, -736.5077) (32.2982, -736.5818) knots 0 0 0 0 0.035532 0.069798 0.069798 0.069798 0.069798
  spline S942 degree 3 poles (32.2982, -736.5818) (32.2249, -736.6885) (32.0578, -736.9317) (32.0501, -737.2286) (32.0459, -737.3953) knots 0 0 0 0 0.038079 0.086792 0.086792 0.086792 0.086792
  line L662 (32.0459, -737.3953) -> (32.0459, -739.4996)
  line L663 (32.0459, -739.4996) -> (31.432, -739.4997)
  line L664 (31.432, -739.4997) -> (31.4319, -737.1463)
  spline S943 degree 3 poles (31.4319, -737.1463) (31.4295, -737.0243) (31.4252, -736.8075) (31.3254, -736.6161) (31.2818, -736.5324) knots 0 0 0 0 0.036008 0.063954 0.063954 0.063954 0.063954
  spline S944 degree 3 poles (31.2818, -736.5324) (31.2196, -736.4728) (31.0834, -736.3424) (30.8937, -736.3329) (30.7907, -736.3278) knots 0 0 0 0 0.025037 0.054812 0.054812 0.054812 0.054812
  spline S945 degree 3 poles (30.7907, -736.3278) (30.706, -736.3335) (30.5365, -736.3448) (30.3865, -736.4244) (30.3115, -736.4642) knots 0 0 0 0 0.025172 0.050327 0.050327 0.050327 0.050327
  spline S946 degree 3 poles (30.3115, -736.4642) (30.2429, -736.5159) (30.1026, -736.6215) (30.0298, -736.7815) (29.9926, -736.8633) knots 0 0 0 0 0.025339 0.051812 0.051812 0.051812 0.051812
  spline S947 degree 3 poles (29.9926, -736.8633) (29.9639, -736.9696) (29.8971, -737.2171) (29.895, -737.4739) (29.8937, -737.6204) knots 0 0 0 0 0.032907 0.076633 0.076633 0.076633 0.076633
  line L665 (29.8937, -737.6204) -> (29.8938, -739.4997)
  line L666 (29.8938, -739.4997) -> (29.2799, -739.4997)
  line L667 (20.1598, -739.4999) -> (19.5459, -739.4999)
  line L668 (19.5459, -739.4999) -> (19.5458, -735.5879)
  spline S948 degree 3 poles (19.5458, -735.5879) (19.4621, -735.6608) (19.2807, -735.8186) (19.0751, -735.9436) (18.9643, -736.0109) knots 0 0 0 0 0.033221 0.072019 0.072019 0.072019 0.072019
  spline S949 degree 3 poles (18.9643, -736.0109) (18.8518, -736.0753) (18.6431, -736.1948) (18.4206, -736.286) (18.318, -736.3281) knots 0 0 0 0 0.03884 0.072064 0.072064 0.072064 0.072064
  line L669 (18.318, -736.3281) -> (18.318, -735.7346)
  spline S950 degree 3 poles (18.318, -735.7346) (18.4826, -735.6511) (18.804, -735.488) (19.0825, -735.2595) (19.2184, -735.148) knots 0 0 0 0 0.05519 0.10775 0.10775 0.10775 0.10775
  spline S951 degree 3 poles (19.2184, -735.148) (19.3344, -735.0399) (19.5471, -734.8418) (19.6962, -734.5927) (19.7641, -734.4795) knots 0 0 0 0 0.047275 0.086674 0.086674 0.086674 0.086674
  line L670 (19.7641, -734.4795) -> (20.1597, -734.4795)
  line L671 (20.1597, -734.4795) -> (20.1598, -739.4999)
  line L672 (28.5502, -789.465) -> (28.5499, -785.8429)
  line L673 (28.5499, -785.8429) -> (29.0991, -785.8429)
  line L674 (29.0991, -785.8429) -> (29.0991, -786.3511)
  spline S952 degree 3 poles (29.0991, -786.3511) (29.161, -786.2665) (29.2859, -786.096) (29.4633, -785.981) (29.5527, -785.923) knots 0 0 0 0 0.031158 0.062835 0.062835 0.062835 0.062835
  spline S953 degree 3 poles (29.5527, -785.923) (29.6519, -785.8758) (29.8557, -785.7786) (30.0814, -785.767) (30.1973, -785.761) knots 0 0 0 0 0.032617 0.067048 0.067048 0.067048 0.067048
  spline S954 degree 3 poles (30.1973, -785.761) (30.3218, -785.7657) (30.5542, -785.7745) (30.7612, -785.8794) (30.8572, -785.928) knots 0 0 0 0 0.036859 0.068796 0.068796 0.068796 0.068796
  spline S955 degree 3 poles (30.8572, -785.928) (30.9369, -785.9898) (31.0979, -786.1144) (31.1794, -786.301) (31.2205, -786.3953) knots 0 0 0 0 0.029725 0.060035 0.060035 0.060035 0.060035
  spline S956 degree 3 poles (31.2205, -786.3953) (31.3707, -786.2103) (31.6618, -785.8517) (32.1182, -785.7905) (32.3392, -785.7608) knots 0 0 0 0 0.068625 0.133023 0.133023 0.133023 0.133023
  spline S957 degree 3 poles (32.3392, -785.7608) (32.5042, -785.7692) (32.8121, -785.7849) (33.0552, -785.9723) (33.168, -786.0592) knots 0 0 0 0 0.048244 0.08997 0.08997 0.08997 0.08997
  spline S958 degree 3 poles (33.168, -786.0592) (33.2523, -786.1815) (33.4417, -786.4564) (33.4522, -786.792) (33.4579, -786.9783) knots 0 0 0 0 0.043695 0.098195 0.098195 0.098195 0.098195
  line L675 (33.4579, -786.9783) -> (33.4581, -789.4647)
  line L676 (33.4581, -789.4647) -> (32.8476, -789.4647)
  line L677 (32.8476, -789.4647) -> (32.8475, -787.183)
  spline S959 degree 3 poles (32.8475, -787.183) (32.8474, -787.0768) (32.8474, -786.8975) (32.805, -786.7235) (32.7877, -786.6526) knots 0 0 0 0 0.031711 0.053535 0.053535 0.053535 0.053535
  spline S960 degree 3 poles (32.7877, -786.6526) (32.7633, -786.601) (32.7134, -786.4956) (32.6192, -786.4268) (32.5711, -786.3918) knots 0 0 0 0 0.016863 0.034394 0.034394 0.034394 0.034394
  spline S961 degree 3 poles (32.5711, -786.3918) (32.5154, -786.3629) (32.4, -786.3032) (32.27, -786.2964) (32.2028, -786.2929) knots 0 0 0 0 0.018597 0.038532 0.038532 0.038532 0.038532
  spline S962 degree 3 poles (32.2028, -786.2929) (32.0816, -786.3027) (31.8437, -786.3219) (31.6591, -786.4729) (31.5684, -786.547) knots 0 0 0 0 0.035532 0.069798 0.069798 0.069798 0.069798
  spline S963 degree 3 poles (31.5684, -786.547) (31.4951, -786.6537) (31.328, -786.8969) (31.3204, -787.1938) (31.3161, -787.3605) knots 0 0 0 0 0.038079 0.086792 0.086792 0.086792 0.086792
  line L678 (31.3161, -787.3605) -> (31.3162, -789.4648)
  line L679 (31.3162, -789.4648) -> (30.7023, -789.4649)
  line L680 (30.7023, -789.4649) -> (30.7022, -787.1115)
  spline S964 degree 3 poles (30.7022, -787.1115) (30.6997, -786.9895) (30.6954, -786.7727) (30.5956, -786.5813) (30.552, -786.4976) knots 0 0 0 0 0.036008 0.063954 0.063954 0.063954 0.063954
  spline S965 degree 3 poles (30.552, -786.4976) (30.4898, -786.4381) (30.3536, -786.3077) (30.1639, -786.2982) (30.0609, -786.293) knots 0 0 0 0 0.025037 0.054812 0.054812 0.054812 0.054812
  spline S966 degree 3 poles (30.0609, -786.293) (29.9761, -786.2987) (29.8067, -786.3101) (29.6567, -786.3897) (29.5817, -786.4295) knots 0 0 0 0 0.025172 0.050327 0.050327 0.050327 0.050327
  spline S967 degree 3 poles (29.5817, -786.4295) (29.5131, -786.4812) (29.3728, -786.5868) (29.3, -786.7468) (29.2628, -786.8286) knots 0 0 0 0 0.025339 0.051812 0.051812 0.051812 0.051812
  spline S968 degree 3 poles (29.2628, -786.8286) (29.2341, -786.9349) (29.1673, -787.1824) (29.1652, -787.4392) (29.164, -787.5857) knots 0 0 0 0 0.032907 0.076633 0.076633 0.076633 0.076633
  line L681 (29.164, -787.5857) -> (29.1641, -789.465)
  line L682 (29.1641, -789.465) -> (28.5502, -789.465)
  line L683 (27.416, -838.1729) -> (28.0197, -838.2513)
  spline S969 degree 3 poles (28.0197, -838.2513) (27.9771, -838.4452) (27.8953, -838.817) (27.6369, -839.0953) (27.5133, -839.2285) knots 0 0 0 0 0.058356 0.111856 0.111856 0.111856 0.111856
  spline S970 degree 3 poles (27.5133, -839.2285) (27.3672, -839.3314) (27.0671, -839.5429) (26.7004, -839.5684) (26.5123, -839.5815) knots 0 0 0 0 0.052559 0.107965 0.107965 0.107965 0.107965
  spline S971 degree 3 poles (26.5123, -839.5815) (26.2792, -839.564) (25.8276, -839.5301) (25.4834, -839.2373) (25.3168, -839.0956) knots 0 0 0 0 0.068154 0.132052 0.132052 0.132052 0.132052
  spline S972 degree 3 poles (25.3168, -839.0956) (25.1853, -838.9048) (24.8974, -838.4874) (24.8763, -837.9786) (24.8649, -837.7023) knots 0 0 0 0 0.068157 0.149141 0.149141 0.149141 0.149141
  spline S973 degree 3 poles (24.8649, -837.7023) (24.8712, -837.5171) (24.8832, -837.1646) (25.0026, -836.833) (25.0592, -836.6757) knots 0 0 0 0 0.055211 0.105055 0.105055 0.105055 0.105055
  spline S974 degree 3 poles (25.0592, -836.6757) (25.1314, -836.5388) (25.2736, -836.2692) (25.5265, -836.0993) (25.651, -836.0157) knots 0 0 0 0 0.04564 0.089884 0.089884 0.089884 0.089884
  spline S975 degree 3 poles (25.651, -836.0157) (25.7869, -835.9516) (26.0608, -835.8223) (26.3632, -835.8046) (26.5156, -835.7957) knots 0 0 0 0 0.044643 0.089955 0.089955 0.089955 0.089955
  spline S976 degree 3 poles (26.5156, -835.7957) (26.6993, -835.8051) (27.0472, -835.8228) (27.3418, -836.0071) (27.4808, -836.0941) knots 0 0 0 0 0.054149 0.102527 0.102527 0.102527 0.102527
  spline S977 degree 3 poles (27.4808, -836.0941) (27.5953, -836.2076) (27.8343, -836.4446) (27.9181, -836.7714) (27.9617, -836.9416) knots 0 0 0 0 0.047449 0.099081 0.099081 0.099081 0.099081
  line L684 (27.9617, -836.9416) -> (27.3648, -837.0337)
  spline S978 degree 3 poles (27.3648, -837.0337) (27.334, -836.9224) (27.2765, -836.7149) (27.1306, -836.5575) (27.063, -836.4846) knots 0 0 0 0 0.034086 0.063475 0.063475 0.063475 0.063475
  spline S979 degree 3 poles (27.063, -836.4846) (26.986, -836.4309) (26.8287, -836.3212) (26.6372, -836.3075) (26.5394, -836.3005) knots 0 0 0 0 0.027619 0.056426 0.056426 0.056426 0.056426
  spline S980 degree 3 poles (26.5394, -836.3005) (26.3928, -836.3135) (26.1037, -836.3393) (25.8907, -836.5361) (25.7857, -836.6331) knots 0 0 0 0 0.04285 0.084486 0.084486 0.084486 0.084486
  spline S981 degree 3 poles (25.7857, -836.6331) (25.7015, -836.7726) (25.5077, -837.0941) (25.5001, -837.4716) (25.4958, -837.6852) knots 0 0 0 0 0.048123 0.11083 0.11083 0.11083 0.11083
  spline S982 degree 3 poles (25.4958, -837.6852) (25.4994, -837.901) (25.5057, -838.2797) (25.6944, -838.6057) (25.7755, -838.7459) knots 0 0 0 0 0.063398 0.111295 0.111295 0.111295 0.111295
  spline S983 degree 3 poles (25.7755, -838.7459) (25.8767, -838.8424) (26.0813, -839.0376) (26.363, -839.0636) (26.5054, -839.0768) knots 0 0 0 0 0.040675 0.082263 0.082263 0.082263 0.082263
  spline S984 degree 3 poles (26.5054, -839.0768) (26.6198, -839.0685) (26.8427, -839.0525) (27.0219, -838.9197) (27.1091, -838.855) knots 0 0 0 0 0.033628 0.065508 0.065508 0.065508 0.065508
  spline S985 degree 3 poles (27.1091, -838.855) (27.1832, -838.7651) (27.3466, -838.5664) (27.3915, -838.312) (27.416, -838.1729) knots 0 0 0 0 0.034396 0.07593 0.07593 0.07593 0.07593
  spline S986 degree 3 poles (19.0565, -837.034) (19.0601, -836.7657) (19.0666, -836.2825) (19.1859, -835.8147) (19.2389, -835.6067) knots 0 0 0 0 0.080152 0.144341 0.144341 0.144341 0.144341
  spline S987 degree 3 poles (19.2389, -835.6067) (19.3036, -835.4398) (19.4261, -835.1233) (19.6672, -834.8853) (19.7812, -834.7728) knots 0 0 0 0 0.052977 0.10048 0.10048 0.10048 0.10048
  spline S988 degree 3 poles (19.7812, -834.7728) (19.9126, -834.6872) (20.1874, -834.5083) (20.5155, -834.4893) (20.6867, -834.4794) knots 0 0 0 0 0.046203 0.096661 0.096661 0.096661 0.096661
  spline S989 degree 3 poles (20.6867, -834.4794) (20.8145, -834.485) (21.06, -834.4957) (21.2849, -834.5942) (21.3927, -834.6414) knots 0 0 0 0 0.037989 0.072993 0.072993 0.072993 0.072993
  spline S990 degree 3 poles (21.3927, -834.6414) (21.49, -834.7021) (21.6873, -834.8253) (21.8245, -835.0133) (21.8941, -835.1086) knots 0 0 0 0 0.034048 0.069103 0.069103 0.069103 0.069103
  spline S991 degree 3 poles (21.8941, -835.1086) (21.9574, -835.2196) (22.0914, -835.4545) (22.1655, -835.7148) (22.2045, -835.8521) knots 0 0 0 0 0.038176 0.080832 0.080832 0.080832 0.080832
  spline S992 degree 3 poles (22.2045, -835.8521) (22.2372, -836.0232) (22.3118, -836.4133) (22.3152, -836.8108) (22.3171, -837.0339) knots 0 0 0 0 0.052146 0.118926 0.118926 0.118926 0.118926
  spline S993 degree 3 poles (22.3171, -837.0339) (22.3135, -837.3005) (22.3069, -837.7813) (22.1889, -838.247) (22.1364, -838.4545) knots 0 0 0 0 0.079639 0.143634 0.143634 0.143634 0.143634